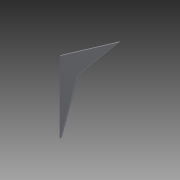
# Autodesk Inventor part: Left Hip
Saved by Autodesk Inventor 2014 (Build 180170000, 170)
## iProperties
Created: 2015-08-01
Part Number: Left Hip
Material: Generic
Document SubType Name: Modeling
Designer: Devon
Density: 1 g/cm^3
Appearance: Default
Author: Devon
Autodesk Inventor part; units mm, degrees
ref_plane "YZ Plane" through (0, 0, 0) normal (1, 0, 0) x (0, 1, 0)
ref_plane "XZ Plane" through (0, 0, 0) normal (0, 1, 0) x (-1, 0, 0)
ref_plane "XY Plane" through (0, 0, 0) normal (0, 0, 1) x (1, 0, 0)
sketch "Sketch1" plane through (0, 0, 0) normal (0, 0, 1) x (1, 0, 0)
  line L0 (2.2943, 2.9258) -> (2.2943, -105.0242)
  line L1 (2.2943, 2.9258) -> (90.7218, 64.8434)
  line L2 (90.7218, 64.8434) -> (27.6787, -10.2885)
  line L3 (2.2943, -105.0242) -> (27.6787, -10.2885)
  point P0 (0, 0)
  dimension "d0" = 107.95
  dimension "d1" = 107.95
  constraints: 8 end point, 1 vertical
  measures "d0" distance of L0.start L0.end
  measures "d1" distance of L0.start L1.end
extrude "Extrusion1" add sketch "Sketch1" along normal blind 3.175
body "Solid1"
